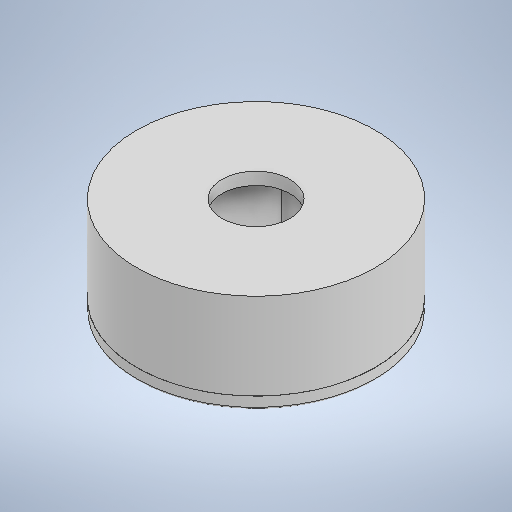
# Autodesk Inventor part: NutRetainer
Saved by Autodesk Inventor 2026 (Build 300175050, 175E)
## iProperties
Created: 2026-02-17
Part Number: NutRetainer
Material: Generic
Document SubType Name: Modeling
Designer: Cupri
Density: 1 g/cm^3
Appearance: Default
Author: Cupri
Autodesk Inventor part; units mm, degrees
ref_plane "YZ Plane" through (0, 0, 0) normal (1, 0, 0) x (0, 1, 0)
ref_plane "XZ Plane" through (0, 0, 0) normal (0, 1, 0) x (-1, 0, 0)
ref_plane "XY Plane" through (0, 0, 0) normal (0, 0, 1) x (1, 0, 0)
sketch "Sketch1" plane through (0, 0, 0) normal (0, 1, 0) x (-1, 0, 0)
  circle A0 centre (0, 0) radius 9.625
  circle A1 centre (0, 0) radius 7.7
  dimension "d0" = 19.25
  dimension "d1" = 15.4
  constraints: 2 centre point, 2 coincident
  measures "d0" diameter of A0
  measures "d1" diameter of A1
extrude "Extrusion1" add sketch "Sketch1" along normal blind 1
sketch "Sketch2" plane through (0, 1, 0) normal (0, 1, 0) x (1, 0, 0)
  circle A0 centre (0, 0) radius 9.6436
  line L0 (-2.8579, 4.95) -> (2.8579, 4.95)
  line L1 (2.8579, 4.95) -> (5.7158, 0)
  line L2 (5.7158, 0) -> (2.8579, -4.95)
  line L3 (2.8579, -4.95) -> (-2.8579, -4.95)
  line L4 (-2.8579, -4.95) -> (-5.7158, 0)
  line L5 (-5.7158, 0) -> (-2.8579, 4.95)
  line L6 (0, 0) -> (0, -3.104)
  line L7 (0, 0) -> (3.104, 0) construction
  dimension "d4" = 9.9
  dimension "d5" = 90
  constraints: 16 end point, 2 coincident, 2 perpendicular, 1 centre point, 1 horizontal, 13 other
  measures "d4" distance between parallel lines of L0 L3
  measures "d5" angle of L6 L7
extrude "Extrusion2" add sketch "Sketch2" along normal blind 6
sketch "Sketch3" plane through (0, 7, 0) normal (0, 1, 0) x (1, 0, 0)
  circle A0 centre (0, 0) radius 9.6436
  circle A1 centre (0, 0) radius 2.75
  circle A2 centre (0, 0) radius 9.6436 projected
  dimension "d8" = 5.5
  dimension "d9" = 0
  constraints: 2 centre point, 2 coincident
  measures "d8" diameter of A1
  measures "d9" radial gap between concentric circles of A2 A0
extrude "Extrusion3" add sketch "Sketch3" along normal blind 1
fillet "Fillet1" radius 0.2 2 edges at (9.625, 0, 0) (7.7, 0, 0)
body "Solid1"
